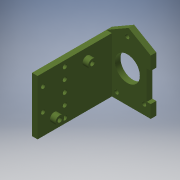
# Autodesk Inventor part: motor mount 2
Saved by Autodesk Inventor 2018 (Build 220112000, 112)
## iProperties
Created: 2017-11-21
Part Number: motor mount 2
Material: ABS Plastic
Document SubType Name: Modeling
Designer: prakhar
Density: 1.06 g/cm^3
Appearance: Olive Green
Author: prakhar
Autodesk Inventor part; units mm, degrees
ref_plane "YZ Plane" through (0, 0, 0) normal (1, 0, 0) x (0, 1, 0)
ref_plane "XZ Plane" through (0, 0, 0) normal (0, 1, 0) x (-1, 0, 0)
ref_plane "XY Plane" through (0, 0, 0) normal (0, 0, 1) x (1, 0, 0)
sketch "Sketch1" plane through (0, 0, 0) normal (1, 0, 0) x (0, 1, 0)
  line L0 (19.8793, 20.7795) -> (-17.4785, 20.7795)
  line L1 (-17.4785, 20.7795) -> (-17.4785, -16.5784)
  line L2 (-17.4785, -16.5784) -> (19.8793, -16.5784)
  line L3 (19.8793, -16.5784) -> (19.8793, 20.7795)
  circle A0 centre (19.8793, 20.7795) radius 4.8895
  circle A1 centre (19.8793, -16.5784) radius 4.8895
  circle A2 centre (-17.4785, -16.5784) radius 4.8895
  circle A3 centre (-17.4785, 20.7795) radius 4.8895
  line L4 (32.5793, 39.8295) -> (-30.1785, 39.8295)
  line L5 (-30.1785, 39.8295) -> (-30.1785, -45.1534)
  line L6 (-30.1785, -45.1534) -> (32.5793, -45.1534)
  line L7 (32.5793, -45.1534) -> (32.5793, 39.8295)
  circle A4 centre (19.8793, 20.7795) radius 2.4575
  circle A5 centre (19.8793, -16.5784) radius 2.4575
  circle A6 centre (-17.4785, -16.5784) radius 2.4575
  circle A7 centre (-17.4785, 20.7795) radius 2.4575
  point P0 (0, 0)
  dimension "d0" = 9.779
  dimension "d4" = 52.832
  dimension "d5" = 12.7
  dimension "d6" = 19.05
  dimension "d7" = 12.7
  dimension "d8" = 28.575
  dimension "d13" = 4.9149
  constraints: 16 end point, 8 centre point, 8 coincident, 6 equal radius, 4 parallel, 3 perpendicular, 2 horizontal
  measures "d0" diameter of A2
  measures "d4" distance of L2.end L0.end
  measures "d5" distance from line of L0.end L5
  measures "d6" distance between parallel lines of L4 L0
  measures "d7" distance between parallel lines of L7 L3
  measures "d8" distance between parallel lines of L6 L2
  measures "d13" diameter of A4
extrude "Extrusion1" add sketch "Sketch1" along normal blind 6.35 contours A3 L1 A7 L0 | L0 A7 L1 A3 | L0 A0 L3 A1 L2 A2 L1 A3 | A7 L1 L0 | L0 L1 A7 | A0 L3 A4 L0 | L0 A4 L3 A0 | A4 L3 L0 | L0 L3 A4 | A2 L2 A6 L1 | L1 A6 L2 A2 | A1 L2 A5 L3 | L3 A5 L2 A1 | A6 L2 L1 | L1 L2 A6 | A5 L2 L3 | L3 L2 A5 | L7 L6 L5 L4
extrude "Extrusion2" add sketch "Sketch1" along normal blind 12.7 contours A3 L1 A7 L0 | L0 A7 L1 A3 | A7 L1 L0 | L0 L1 A7 | A1 L2 A5 L3 | L3 A5 L2 A1 | A5 L2 L3 | L3 L2 A5
extrude "Extrusion3" cut sketch "Sketch1" along normal blind 12.7 contours A7 L1 L0 | L0 L1 A7 | A5 L2 L3 | L3 L2 A5
sketch "Sketch2" plane through (0, -30.1785, -45.1534) normal (0, 0, -1) x (-1, 0, 0)
  line L0 (0, 0) -> (-6.35, 0) projected
  line L1 (0, 0) -> (-50.8, 0)
  line L2 (-50.8, 0) -> (-50.8, 62.7579)
  line L3 (-50.8, 62.7579) -> (0, 62.7579)
  line L4 (0, 62.7579) -> (0, 0)
  line L5 (0, 62.7579) -> (-6.35, 62.7579) projected
  line L6 (-50.8, 62.7579) -> (-25.4, 77.4226)
  line L7 (-25.4, 77.4226) -> (0, 62.7579)
  line L8 (-50.8, 62.7579) -> (0, 62.7579)
  point P0 (0, 30.1785)
  dimension "d16" = 50.8
  dimension "d89" = 30
  dimension "d90" = 30
  constraints: 14 end point, 2 parallel, 1 collinear, 1 horizontal, 1 perpendicular
  measures "d16" distance of L2.end L3.end
  measures "d89" angle of L3 L7
  measures "d90" angle of L3 L6
extrude "Extrusion4" add sketch "Sketch2" along normal blind 6.35
sketch "Sketch4" plane through (0, 32.5793, 39.8295) normal (0, 1, 0) x (1, 0, 0)
  line L0 (0, 84.9829) -> (0, 0) projected
  line L1 (0, 0) -> (6.35, 0) projected
  line L2 (6.35, 84.9829) -> (6.35, 0) projected
  line L3 (0, 78.6329) -> (6.35, 78.6329)
  line L4 (6.35, 78.6329) -> (6.35, 129.4329)
  line L5 (6.35, 129.4329) -> (0, 129.4329)
  line L6 (0, 129.4329) -> (0, 78.6329)
  line L7 (6.35, 129.4329) -> (50.8, 129.4329)
  line L8 (50.8, 129.4329) -> (50.8, 123.0829)
  line L9 (50.8, 123.0829) -> (6.35, 123.0829)
  line L10 (6.35, 123.0829) -> (6.35, 129.4329)
  line L11 (0, 84.9829) -> (6.35, 84.9829) projected
  point P0 (0, 39.8295)
  dimension "d25" = 6.35
  dimension "d26" = 50.8
  dimension "d27" = 6.35
  constraints: 16 end point, 4 parallel, 2 horizontal, 2 perpendicular
  measures "d25" distance of L7.end L8.end
  measures "d26" distance of L3.end L4.end
  measures "d27" distance between parallel lines of L6 L4
sketch "Sketch3" plane through (0, -30.1785, -45.1534) normal (0, 0, 1) x (1, 0, 0)
  circle A0 centre (24.1046, 36.4435) radius 9.7536
  line L0 (6.35, 62.7579) -> (6.35, 0) projected
  circle A1 centre (24.1046, 36.4435) radius 14.2494
  line L1 (6.35, 0) -> (50.8, 0) projected
  point P0 (0, 30.1785)
  dimension "d19" = 19.5072
  dimension "d20" = 17.7546
  dimension "d22" = 28.4988
  dimension "d91" = 36.4435
  constraints: 2 centre point, 1 coincident
  measures "d19" diameter of A0
  measures "d20" distance from line of A0.centre L0
  measures "d22" diameter of A1
  measures "d91" distance from line of A0.centre L1
extrude "Extrusion5" cut sketch "Sketch3" against normal blind 63.5 contours A0 | A1
sketch "Sketch5" plane through (0, -30.1785, -45.1534) normal (0, 0, 1) x (1, 0, 0)
  circle A0 centre (24.1046, 36.4435) radius 14.2494 projected
  circle A1 centre (23.8385, 68.1924) radius 2.4574
  circle A2 centre (43.1546, 11.0435) radius 2.4574
  circle A3 centre (11.6326, 7.2457) radius 2.4574
  point P0 (0, 30.1785)
  dimension "d33" = 4.9149
  dimension "d46" = 31.75
  dimension "d47" = 31.75
  dimension "d48" = 31.75
  dimension "d49" = 31.75
  dimension "d50" = 60.325
  dimension "d51" = 25.4
  constraints: 3 centre point, 2 equal radius
  measures "d33" diameter of A2
  measures "d46" distance of A0.centre A1.centre
  measures "d47" distance of A0.centre A2.centre
  measures "d48" distance of A0.centre A3.centre
  measures "d49" distance of A2.centre A3.centre
  measures "d50" distance of A1.centre A2.centre
  measures "d51" vertical distance of A0.centre A2.centre
extrude "Extrusion7" cut sketch "Sketch5" against normal blind 25.4 contours A1 | A2 | A3
ref_plane "Work Plane1" through (-9.525, -30.1785, 2.2051) normal (-1, 0, 0) x (0, 0, 1)
sketch "Sketch10" plane through (0, 0, 0) normal (-1, 0, 0) x (0, 0, 1)
  line L0 (14.9051, -30.1785) -> (14.9051, 32.5793) projected
  line L1 (14.9051, 32.5793) -> (2.2051, 32.5793) projected
  circle A0 centre (8.5551, 26.2293) radius 2.4574
  circle A1 centre (8.5551, 13.5293) radius 2.4574
  circle A2 centre (8.5551, 0.8293) radius 2.4574
  circle A3 centre (8.5551, -11.8707) radius 2.4574
  circle A4 centre (8.5551, -24.5707) radius 2.4574
  point P0 (0, 0)
  dimension "d77" = 4.9149
  dimension "d78" = 6.35
  dimension "d79" = 6.35
  dimension "d82" = 12.7
  constraints: 5 centre point, 1 vertical, 8 other
  measures "d77" diameter of A0
  measures "d78" distance from line of L0 A0.centre
  measures "d79" distance from line of A0.centre L1
  measures "d82" distance of A0.centre A1.centre
extrude "Extrusion12" cut sketch "Sketch10" against normal blind 25.4
sketch "Sketch11" plane through (0, -30.1785, -45.1534) normal (0, 0, 1) x (1, 0, 0)
  line L0 (52.0296, 47.0435) -> (52.0296, 15.1435)
  line L1 (46.7796, 15.1435) -> (46.7796, 47.0435)
  line L2 (52.0296, 15.1435) -> (46.7796, 15.1435)
  line L3 (46.7796, 47.0435) -> (52.0296, 47.0435)
  line L4 (46.2716, 47.5515) -> (46.2716, 14.6355)
  line L5 (46.2716, 14.6355) -> (52.5376, 14.6355)
  line L6 (52.5376, 14.6355) -> (52.5376, 47.5515)
  line L7 (52.5376, 47.5515) -> (46.2716, 47.5515)
  point P0 (0, 30.1785)
  dimension "d92" = 0.508
  constraints: 16 end point, 4 parallel, 1 horizontal, 5 other
  measures "d92" distance between parallel lines of L1 L4
extrude "Extrusion13" cut sketch "Sketch11" against normal blind 25.4 contours L0 L2 L1 L3 | L7 L6 L5 L4
sketch "Sketch12" plane through (6.35, 0, 0) normal (1, 0, 0) x (0, 0, -1)
  line L0 (51.5034, 20.5143) -> (51.5034, -7.9845) projected
  line L1 (45.1534, -7.9845) -> (45.1534, 20.5143) projected
  line L2 (45.1534, 6.2649) -> (-81.3629, 6.2649)
  circle A0 centre (-33.4795, 18.9649) radius 2.3495
  circle A1 centre (-33.4795, -6.4351) radius 2.3495
  line L3 (-39.8295, 32.5793) -> (-39.8295, -30.1785) projected
  point P0 (0, 0)
  dimension "d95" = 4.699
  dimension "d96" = 4.699
  dimension "d97" = 12.7
  dimension "d98" = 12.7
  dimension "d99" = 6.35
  constraints: 2 centre point, 2 end point, 1 horizontal, 1 midpoint, 1 vertical alignment
  measures "d95" diameter of A0
  measures "d96" diameter of A1
  measures "d97" distance from line of A0.centre L2
  measures "d98" distance from line of L2 A1.centre
  measures "d99" distance from line of A0.centre L3
extrude "Extrusion14" cut sketch "Sketch12" against normal blind 25.4
equation "\"d90\" = d89"
equation "\"d27\" = d25"
equation "\"d1\" = d0"
body "Solid1"
